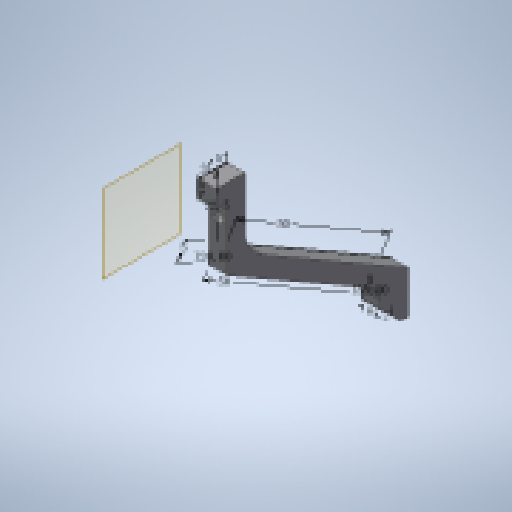
# Autodesk Inventor part: darwin_landing_gear_-_Part_4
Saved by Autodesk Inventor 2025.2 (Build 292293000, 293)
## iProperties
Created: 2025-09-29
Part Number: darwin_landing_gear_-_Part_4
Material: 常规
Document SubType Name: Modeling
Designer: BO‘S_SLAVE
Density: 1 g/cm^3
Appearance: 默认
Author: BO‘S_SLAVE
Autodesk Inventor part; units mm, degrees
ref_plane "YZ Plane" through (0, 0, 0) normal (1, 0, 0) x (0, 1, 0)
ref_plane "XZ Plane" through (0, 0, 0) normal (0, 1, 0) x (-1, 0, 0)
ref_plane "XY Plane" through (0, 0, 0) normal (0, 0, 1) x (1, 0, 0)
ref_plane "工作平面3" through (69, -14.0617, 3) normal (1, 0, 0) x (0, 1, 0)
sketch "草图1" plane through (69, -14.0617, 3) normal (1, 0, 0) x (0, 1, 0)
  line L0 (0, 0) -> (-25, -43.3013)
  line L1 (-22.1132, -48.3013) -> (2.8868, -5)
  line L2 (-30, -43.3013) -> (-35.6569, -48.9581)
  line L3 (-25, -43.3013) -> (-30, -43.3013)
  line L4 (24, 0) -> (24, -5)
  line L5 (-35.6569, -48.9581) -> (-35.6569, -50.9581)
  line L6 (-35.6569, -50.9581) -> (-23.6472, -50.9581)
  line L7 (2.8868, -5) -> (24, -5)
  line L8 (0, 0) -> (24, 0)
  line L9 (24, 0) -> (24, 3)
  line L10 (24, 3) -> (19, 3)
  line L11 (19, 3) -> (19, 0)
  line L12 (-22.1132, -48.3013) -> (-23.6472, -50.9581)
  dimension "d2" = 50
  dimension "d7" = 5
  dimension "d8" = 135
  dimension "d12" = 8
  dimension "d14" = 50
  dimension "d15" = 5
  dimension "d22" = 2
  dimension "d36" = 5
  dimension "d38" = 24
  dimension "d39" = 120
  dimension "d40" = 3
  dimension "d41" = 5
  constraints: 27 end point, 4 horizontal, 4 perpendicular, 1 collinear, 1 parallel, 1 point on line, 1 vertical, 1 other
  measures "d2" distance of L0.start L0.end
  measures "d7" distance between parallel lines of L0 L1
  measures "d8" angle of L2 L3
  measures "d12" distance of L2.start L2.end
  measures "d14" distance of L1.start L1.end
  measures "d15" distance of L0.end L2.start
  measures "d22" distance of L2.end L5.end
  measures "d36" distance of L4.start L4.end
  measures "d38" distance of L0.start L4.start
  measures "d39" angle of L0 L8
  measures "d40" distance of L4.start L9.end
  measures "d41" distance of L9.end L10.end
extrude "拉伸1" add sketch "草图1" along normal blind 5
fillet "圆角2" radius 10 1 edges at (71.5, -11.1749, -2)
fillet "圆角3" radius 5 1 edges at (71.5, -39.0617, -40.3013)
sketch "草图4" plane through (69, -14.0617, 3) normal (0, 0, 1) x (1, 0, 0)
  line L0 (0, 19) -> (0, 0) projected
  line L1 (0, 0) -> (5, 0) projected
  line L2 (5, 19) -> (5, 0) projected
  line L3 (0, 19) -> (5, 19) projected
  circle A0 centre (2.5, 14.5) radius 1.5
  point P0 (-69, 14.0617)
  dimension "d42" = 3
  dimension "d43" = 4.5
  dimension "d44" = 2.5
  constraints: 1 centre point
  measures "d42" diameter of A0
  measures "d43" distance from line of A0.centre L3
  measures "d44" distance from line of L2 A0.centre
extrude "拉伸3" cut sketch "草图4" against normal blind 5 contours A0
